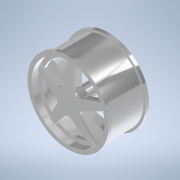
# Autodesk Inventor part: Whell
Saved by Autodesk Inventor 2022.3 (Build 263350000, 350)
## iProperties
Created: 2018-01-08
Part Number: Whell
Material: 알루미늄 6061
Document SubType Name: Modeling
Designer: user
Density: 2.7 g/cm^3
Appearance: 알루미늄 - 평지
Author: user
Autodesk Inventor part; units mm, degrees
ref_plane "YZ Plane" through (0, 0, 0) normal (1, 0, 0) x (0, 1, 0)
ref_plane "XZ Plane" through (0, 0, 0) normal (0, 1, 0) x (-1, 0, 0)
sketch "스케치1" plane through (0, 0, 0) normal (0, 0, 1) x (1, 0, 0)
  circle A0 centre (0, 0) radius 22.5
  circle A1 centre (0, 0) radius 23.5
  dimension "d0" = 45
  dimension "d1" = 1
  dimension "d55" = 47
  constraints: 2 centre point, 2 coincident
  measures "d0" diameter of A0
  measures "d1" radial gap between concentric circles of A1 A0
  measures "d55" diameter of A1
extrude "돌출1" add sketch "스케치1" along normal blind 25
ref_plane "작업 평면1" through (0, 0, 21) normal (0, 0, 1) x (1, 0, 0)
sketch "스케치2" plane through (0, 0, 21) normal (0, 0, 1) x (1, 0, 0)
  circle A0 centre (0, 0) radius 22.5
  circle A1 centre (0, 0) radius 22.5 projected
  circle A2 centre (0, 0) radius 20
  dimension "d5" = 40
  constraints: 2 centre point, 2 coincident, 1 concentric
  measures "d5" diameter of A2
extrude "돌출2" add sketch "스케치2" against normal blind 2
sketch "스케치3" plane through (0, 0, 0) normal (1, 0, 0) x (0, 1, 0)
  line L0 (22.5, 19) -> (-22.5, 19) construction
  line L1 (22.5, 0) -> (22.5, 19) construction
  line L2 (-22.5, 0) -> (-22.5, 19) construction
  line L3 (-22.5, 25) -> (22.5, 25) construction
  line L4 (22.5, 21) -> (22.5, 21.2317)
  arc A0 (21.7533, 22.1991) -> (0, 25) centre (0, -60.875) ccw
  line L5 (-22.5, 21) -> (-22.5, 22) construction
  line L6 (0, 29.0368) -> (0, -29.0368)
  arc A1 (0, 25) -> (-22.5, 22) centre (0, -60.875) ccw construction
  line L7 (-21.5, 21) -> (-21.5, 21.2317) construction
  arc A2 (0, 24) -> (-21.5, 21.2317) centre (0, -60.875) ccw construction
  arc A3 (20.7444, 21.4259) -> (0, 24) centre (0, -60.875) ccw
  line L8 (21.5, 20.4562) -> (21.5, 21)
  line L9 (21.5, 21) -> (22.5, 21)
  line L10 (20, 19) -> (-20, 19) projected
  line L11 (0, 25) -> (0, 24)
  arc A4 (22.5, 21.2317) -> (21.7533, 22.1991) centre (21.5, 21.2317) ccw
  arc A5 (21.5, 20.4562) -> (20.7444, 21.4259) centre (20.5, 20.4562) ccw
  point P0 (0, 0)
  point P1 (22.5, 22)
  point P2 (0, 0)
  point P3 (21.5, 21.2317)
  dimension "d13" = 1
  dimension "d14" = 1
  dimension "d15" = 1
  dimension "d16" = 1
  constraints: 14 end point, 14 point on circle, 6 centre point, 6 tangent, 3 point on line, 3 vertical, 1 coincident, 1 collinear, 1 equal radius, 1 midpoint, 1 parallel, 3 other
  measures "d13" distance of L4.start point (22.5, 22)
  measures "d14" distance of L5.start L5.end
  measures "d15" radial gap between concentric circles of A0 A3
  measures "d16" radius of A4
revolve "회전1" add sketch "스케치3" angle 360 about axis through (0, 0, 29.0368) along (0, 0, -1)
sketch "스케치4" plane through (0, 0, 0) normal (1, 0, 0) x (0, 1, 0)
  line L0 (22.5, 0) -> (22.5, 19) construction
  line L1 (22.5, 14) -> (19.8527, 14)
  line L2 (19.1686, 14.1206) -> (11.5331, 16.8997)
  line L3 (11.4647, 16.9118) -> (0, 16.9118)
  line L4 (0, 16.9118) -> (0, 24.4742)
  line L5 (22.5, 14) -> (22.5, 21.4551)
  line L6 (-21.7533, 22.1991) -> (21.7533, 22.1991) construction
  line L7 (-21.7533, 22.1991) -> (21.7533, 22.1991) construction
  line L8 (22.5, 21.2317) -> (-22.5, 21.2317) construction
  line L9 (22.5, 19) -> (-22.5, 19) construction
  arc A0 (19.1686, 14.1206) -> (19.8527, 14) centre (19.8527, 16) ccw
  arc A1 (11.5331, 16.8997) -> (11.4647, 16.9118) centre (11.4647, 16.7118) ccw
  arc A2 (22.5, 21.4551) -> (0, 24.4742) centre (0, -60.875) ccw
  point P0 (0, 0)
  point P1 (19.5, 14)
  point P2 (11.5, 16.9118)
  point P3 (22.5, 21.2317)
  dimension "d18" = 22.5
  dimension "d20" = 5
  dimension "d21" = 20
  dimension "d22" = 8
  dimension "d23" = 3
  dimension "d24" = 2
  dimension "d25" = 0.2
  constraints: 10 end point, 6 point on circle, 6 point on line, 4 tangent, 3 centre point, 1 collinear, 1 horizontal, 1 parallel, 1 vertical
  measures "d18" distance between parallel lines of L4 L0
  measures "d20" distance between parallel lines of L1 L9
  measures "d21" angle of L1 L2
  measures "d22" horizontal distance of point (19.5, 14) point (11.5, 16.912)
  measures "d23" distance from line of L0 point (19.5, 14)
  measures "d24" radius of A0
  measures "d25" radius of A1
extrude "돌출3" add sketch "스케치4" along normal mid plane 1
pattern_circular "원형 패턴1" count 5 over 360 about axis through (0, 0, 0) along (0, 0, 1) of "돌출3"
sketch "스케치5" plane through (0, 0, 25) normal (0, 0, 1) x (1, 0, 0)
  circle A0 centre (0, 0) radius 22.5 projected
  arc A1 (21.239, 7.4267) -> (0.5, 22.4944) centre (0, 0) ccw projected
  line L0 (1.9423, 22.416) -> (3.1832, 8.2332)
  line L1 (6.8466, 5.5716) -> (20.7187, 8.7742)
  arc A2 (-0.5, 22.4944) -> (-21.239, 7.4267) centre (0, 0) ccw projected
  line L2 (0, 0) -> (0, 32.7756) construction
  line L3 (0, 0) -> (35.7356, 11.6112) construction
  line L4 (0, 0) -> (24.3254, 33.4811) construction
  arc A3 (3.1832, 8.2332) -> (6.8466, 5.5716) centre (6.1717, 8.4947) ccw
  circle A4 centre (0, 0) radius 7.5 construction
  point P0 (3.4839, 4.7952)
  dimension "d31" = 5
  dimension "d33" = 72
  dimension "d34" = 5
  dimension "d35" = 36
  dimension "d36" = 3
  dimension "d37" = 15
  constraints: 10 end point, 6 point on circle, 3 point on line, 3 tangent, 2 centre point, 1 coincident, 1 vertical
  measures "d31" angle of L0 L2
  measures "d33" angle of L2 L3
  measures "d34" angle of L3 L1
  measures "d35" angle of L3 L4
  measures "d36" radius of A3
  measures "d37" diameter of A4
extrude "돌출4" cut sketch "스케치5" against normal up to surface (4 mm away) contours L1 A3 L0 A0 picked at (11.0472, 13.9213)
pattern_circular "원형 패턴2" count 5 over 360 about axis through (0, 0, 0) along (0, 0, 1) of "돌출4"
sketch "스케치6" plane through (0, 0, 25) normal (0, 0, 1) x (1, 0, 0)
  circle A0 centre (0, 0) radius 23.5 projected
  circle A1 centre (0, 0) radius 25
  dimension "d43" = 50
  constraints: 1 centre point, 1 coincident
  measures "d43" diameter of A1
extrude "돌출5" add sketch "스케치6" against normal blind 2
sketch "스케치7" plane through (-0.5, 0.6882, 16.9118) normal (0, 0, -1) x (-1, 0, 0)
  circle A0 centre (-0.5, -0.6882) radius 5
  dimension "d46" = 10
  constraints: 1 centre point, 1 coincident
  measures "d46" diameter of A0
extrude "돌출6" add sketch "스케치7" against normal up to surface draft 20
sketch "스케치8" plane through (0.5, 11.4647, 16.9118) normal (0, 0, -1) x (-1, 0, 0)
  arc A0 (-2.0197, -15.7834) -> (3.0197, -15.7834) centre (0.5, -11.4647) ccw projected
  circle A1 centre (0.5, -11.4647) radius 4
  dimension "d49" = 8
  constraints: 1 centre point, 1 coincident
  measures "d49" diameter of A1
extrude "돌출7" add sketch "스케치8" along normal blind 19
sketch "스케치9" plane through (0, 0, 0) normal (0, 0, -1) x (-1, 0, 0)
  circle A0 centre (0, 0) radius 23.5 projected
  circle A1 centre (0, 0) radius 25
  dimension "d52" = 50
  constraints: 1 centre point, 1 coincident
  measures "d52" diameter of A1
extrude "돌출8" add sketch "스케치9" against normal blind 2
sketch "Sketch10" plane through (0, 0, -2.0882) normal (0, 0, -1) x (-1, 0, 0)
  point P0 (0, 0)
sketch "Sketch11" plane through (0, 0, -2.0882) normal (0, 0, -1) x (-1, 0, 0)
  point P0 (0, 0)
